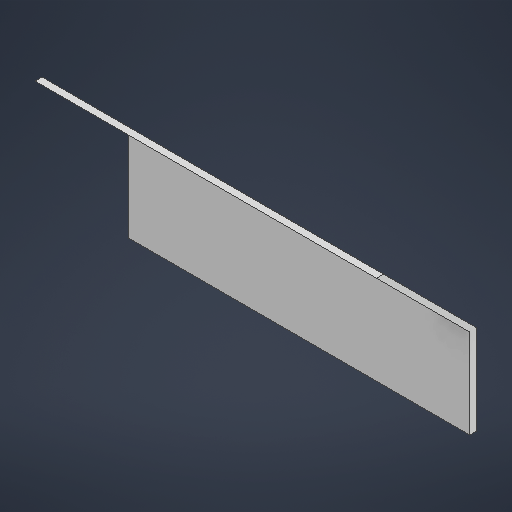
# Autodesk Inventor part: Mini Sumô Definitivo - TAMPA
Saved by Autodesk Inventor 2026.1 (Build 301233000, 233)
## iProperties
Created: 2025-12-03
Part Number: Mini Sumô Definitivo - TAMPA
Material: Genérico
Document SubType Name: Modeling
Designer: panto
Density: 1 g/cm^3
Appearance: Padrão
Author: panto
Autodesk Inventor part; units mm, degrees
ref_plane "YZ Plane" through (0, 0, 0) normal (1, 0, 0) x (0, 1, 0)
ref_plane "XZ Plane" through (0, 0, 0) normal (0, 1, 0) x (-1, 0, 0)
ref_plane "XY Plane" through (0, 0, 0) normal (0, 0, 1) x (1, 0, 0)
sketch "Esboço1" plane through (0, 0, 0) normal (1, 0, 0) x (0, 1, 0)
  line L0 (30.2603, -55.8743) -> (4.9294, -55.8743)
  line L1 (30.2603, -57.9073) -> (4.9294, -57.9073)
  line L2 (56.7603, -29.3743) -> (30.2603, -55.8743)
  line L3 (56.7603, -31.3743) -> (30.2603, -57.9073)
  line L4 (4.9294, -55.8743) -> (4.9294, -57.9073)
  line L5 (56.7603, -29.3743) -> (56.7603, -31.3743)
  point P0 (0, 0)
  point P1 (56.7603, -55.8743)
  point P2 (56.7603, -55.8743)
  dimension "d4" = 26.5
  dimension "d5" = 26.5
  dimension "d6" = 2
  dimension "d7" = 37.5
  constraints: 12 end point, 2 point on line, 2 vertical
  measures "d4" distance of L2.start point (56.76, -55.874)
  measures "d5" distance of L0.start point (56.76, -55.874)
  measures "d6" distance of L2.start L3.start
  measures "d7" distance of L3.start L1.start
extrude "Extrusão1" add sketch "Esboço1" along normal blind 97
equation "\"d5\" = d4"
